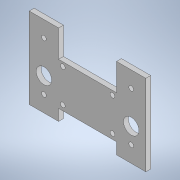
# Autodesk Inventor part: gps_plate
Saved by Autodesk Inventor 2021 (Build 250183000, 183)
## iProperties
Created: 2020-12-14
Part Number: gps_plate
Material: Generic
Document SubType Name: Modeling
Designer: Mateusz
Density: 1 g/cm^3
Appearance: Default
Author: Mateusz
Autodesk Inventor part; units mm, degrees
ref_plane "YZ Plane" through (0, 0, 0) normal (1, 0, 0) x (0, 1, 0)
ref_plane "Work Plane1" through (0, 0, 0) normal (0, 0, 1) x (1, 0, 0)
sketch "Sketch1" plane through (0, 0, 0) normal (0, 0, 1) x (1, 0, 0)
  line L0 (0, -26.08) -> (0, 0) projected
  line L1 (35.6, -26.08) -> (0, -26.08) projected
  line L2 (35.6, 0) -> (35.6, -26.08) projected
  line L3 (0, 0) -> (35.6, 0) projected
  point P0 (33.1, -3.1792)
  point P1 (33.1, -23.5192)
  point P2 (2.6, -23.48)
  point P3 (2.6, -3.14)
extrude "Extrusion1" add sketch "Sketch1" along normal blind 3
sketch "Sketch2" plane through (0, 0, 0) normal (0, 0, -1) x (-1, 0, 0)
  line L0 (-49.6, 16.67) -> (-39.6, 16.67) projected
  line L1 (-39.6, 16.67) -> (-35.6, 16.67) projected
  line L2 (-49.6, 16.67) -> (-53.6, 16.67) projected
  line L3 (-50.6, -33.042) -> (-53.6, -33.042) projected
  line L4 (-38.6, -33.042) -> (-35.6, -33.042) projected
  line L5 (4, 16.67) -> (0, 16.67) projected
  line L6 (4, 16.67) -> (14, 16.67) projected
  line L7 (14, 16.67) -> (18, 16.67) projected
  line L8 (15, -33.042) -> (18, -33.042) projected
  line L9 (3, -33.042) -> (0, -33.042) projected
  line L10 (0, 16.67) -> (0, -33.042) projected
  line L11 (-35.6, -33.042) -> (-35.6, 16.67) projected
  circle A0 centre (-44.6, 6.817) radius 1.45 projected
  circle A1 centre (-44.6001, -23.183) radius 1.4501 projected
  circle A2 centre (9, -23.183) radius 1.45 projected
  circle A3 centre (9, 6.817) radius 1.45 projected
  line L12 (-53.6, 16.67) -> (-53.6, -33.042) projected
  line L13 (-35.6, -26.08) -> (-35.6, 0) projected
  line L14 (-35.6, 0) -> (-35.6, -26.08)
  line L15 (-38.6, -33.042) -> (-50.6, -33.042)
  line L16 (3, -33.042) -> (15, -33.042)
  line L17 (18, -33.042) -> (18, 16.67)
  point P0 (0, 0)
  constraints: 8 end point, 2 horizontal, 1 collinear, 1 perpendicular
ref_plane "Work Plane2" through (0, -26.08, 3) normal (0, 0, -1) x (0, 1, 0)
extrude "Extrusion2" add sketch "Sketch2" against normal up to surface (3 mm away)
sketch "Sketch3" plane through (0, 0, 3) normal (0, 0, 1) x (1, 0, 0)
  circle A0 centre (2.6, -22.94) radius 1.6 projected
  circle A1 centre (33.1, -22.9008) radius 1.6 projected
  circle A2 centre (33.1, -2.5608) radius 1.6 projected
  circle A3 centre (2.6, -2.6) radius 1.6 projected
  circle A4 centre (2.6, -2.6) radius 1.45
  circle A5 centre (2.6, -22.94) radius 1.45
  circle A6 centre (33.1, -22.9008) radius 1.45
  circle A7 centre (33.1, -2.5608) radius 1.45
  point P0 (0, 0)
  dimension "d8" = 2.9
  dimension "d9" = 2.9
  dimension "d10" = 2.9
  dimension "d11" = 2.9
  constraints: 4 centre point, 4 coincident
  measures "d8" diameter of A4
  measures "d9" diameter of A5
  measures "d10" diameter of A6
  measures "d11" diameter of A7
extrude "Extrusion3" cut sketch "Sketch3" against normal through all contours A4 | A5 | A6 | A7
sketch "Sketch4" plane through (0, 0, 3) normal (0, 0, 1) x (1, 0, 0)
  circle A0 centre (-9, -23.183) radius 1.45 projected
  line L0 (-9, -23.183) -> (-9, -13.251)
  circle A1 centre (-9, -13.251) radius 4.767
  circle A2 centre (44.6001, -23.183) radius 1.4501 projected
  line L1 (44.6001, -23.183) -> (44.6001, -13.251)
  circle A3 centre (44.6001, -13.251) radius 4.767
  point P0 (0, 0)
  dimension "d14" = 9.932
  dimension "d15" = 9.534
  dimension "d16" = 9.534
  constraints: 4 end point, 2 centre point, 2 coincident, 2 vertical
  measures "d14" distance of L0.start L0.end
  measures "d15" diameter of A1
  measures "d16" diameter of A3
extrude "Extrusion4" cut sketch "Sketch4" against normal through all contours A1 | A3
body "Solid1"
